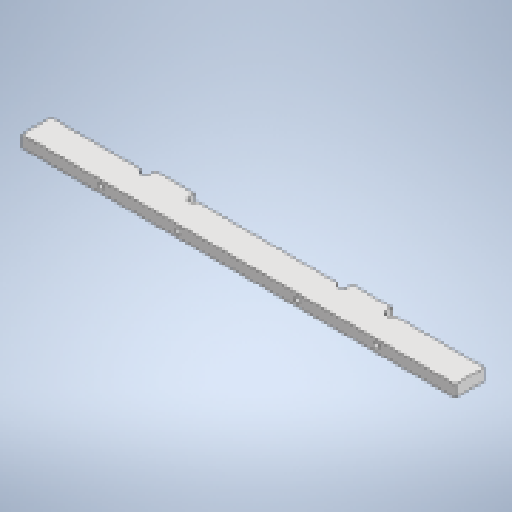
# Autodesk Inventor part: wall
Saved by Autodesk Inventor 2024 (Build 280153000, 153)
## iProperties
Created: 2024-06-06
Part Number: wall
Material: 一般
Document SubType Name: Modeling
Designer: right
Density: 1 g/cm^3
Appearance: 既定
Author: right
Autodesk Inventor part; units mm, degrees
ref_plane "YZ Plane" through (0, 0, 0) normal (1, 0, 0) x (0, 1, 0)
ref_plane "XZ Plane" through (0, 0, 0) normal (0, 1, 0) x (-1, 0, 0)
ref_plane "XY Plane" through (0, 0, 0) normal (0, 0, 1) x (1, 0, 0)
sketch "スケッチ1" plane through (0, 0, 0) normal (0, 0, 1) x (1, 0, 0)
  line L0 (55.5, 22.0883) -> (-55.5, 22.0883)
  line L1 (-55.5, 22.0883) -> (-55.5, 25.0883)
  line L2 (-55.5, 25.0883) -> (55.5, 25.0883)
  line L3 (55.5, 25.0883) -> (55.5, 22.0883)
  line L4 (-22.45, 22.0883) -> (-28.05, 22.0883) projected
  point P0 (0, 0)
  point P1 (-55.5, 26.1052)
  dimension "d0" = 3
  dimension "d1" = 111
  constraints: 8 end point, 2 parallel, 1 horizontal, 1 perpendicular, 1 point on line, 1 vertical alignment, 1 other
  measures "d0" distance of L0.end L1.end
  measures "d1" distance of L1.end L2.end
ref_plane "作業平面1" through (1.2806, -38.0265, 7.5) normal (0, 0, 1) x (0.824865, -0.5653297, 0)
extrude "押し出し1" add sketch "スケッチ1" along normal up to surface (7.5 mm away)
sketch "スケッチ2" plane through (0, 0, 0) normal (0, 0, -1) x (-1, 0, 0)
  line L0 (30.25, 26.1052) -> (30.25, 22.0883) projected
  line L1 (20.25, 22.0883) -> (20.25, 26.1052) projected
  line L2 (-20.25, 26.1052) -> (-20.25, 22.0883) projected
  line L3 (-30.25, 22.0883) -> (-30.25, 26.1052) projected
  line L4 (-55.5, 25.0883) -> (55.5, 25.0883) projected
  line L5 (30.25, 22.0883) -> (20.25, 22.0883)
  line L6 (20.25, 22.0883) -> (20.25, 25.0883)
  line L7 (20.25, 25.0883) -> (30.25, 25.0883)
  line L8 (30.25, 25.0883) -> (30.25, 22.0883)
  line L9 (-20.25, 22.0883) -> (-30.25, 22.0883)
  line L10 (-30.25, 22.0883) -> (-30.25, 25.0883)
  line L11 (-30.25, 25.0883) -> (-20.25, 25.0883)
  line L12 (-20.25, 25.0883) -> (-20.25, 22.0883)
  point P0 (0, 0)
  point P1 (-20.25, 25.0883)
  point P2 (30.25, 25.0883)
  constraints: 16 end point, 4 parallel, 4 point on line, 2 horizontal, 2 perpendicular
ref_plane "作業平面2" through (-55.5, -26.1052, -1.5) normal (0, 0, -1) x (0, 1, 0)
extrude "押し出し2" add sketch "スケッチ2" along normal up to surface (1.5 mm away)
sketch "スケッチ3" plane through (-55.5, 25.0883, 7.5) normal (0, 1, 0) x (1, 0, 0)
  line L0 (85.75, 7.5) -> (111, 7.5) projected
  circle A0 centre (86.85, 7.5) radius 1.1
  line L1 (85.75, 7.5) -> (85.75, 9) projected
  line L2 (75.75, 7.5) -> (35.25, 7.5) projected
  circle A1 centre (74.65, 7.5) radius 1.1
  line L3 (75.75, 7.5) -> (75.75, 9) projected
  line L4 (35.25, 9) -> (35.25, 7.5) projected
  line L5 (25.25, 7.5) -> (25.25, 9) projected
  line L6 (0, 7.5) -> (25.25, 7.5) projected
  circle A2 centre (36.35, 7.5) radius 1.1
  circle A3 centre (24.15, 7.5) radius 1.1
  point P0 (55.5, 7.5)
  dimension "d6" = 2.2
  dimension "d7" = 2.2
  dimension "d8" = 2.2
  dimension "d9" = 2.2
  constraints: 3 horizontal alignment, 3 point on line, 2 vertical, 1 centre point, 1 tangent, 6 other
  measures "d9" diameter of A3
extrude "押し出し3" cut sketch "スケッチ3" against normal through all
sketch "スケッチ4" plane through (0, 0, 0) normal (0, 0, -1) x (-1, 0, 0)
  circle A0 centre (-35.25, 23.5883) radius 1.1 projected
  circle A1 centre (-15.25, 23.5883) radius 1.1 projected
  circle A2 centre (15.25, 23.5883) radius 1.1 projected
  circle A3 centre (35.25, 23.5883) radius 1.1 projected
  point P0 (0, 0)
  constraints: 4 coincident
hole "穴1" at (35.25, 23.5883, 0) at (15.25, 23.5883, 0) at (-15.25, 23.5883, 0) at (-35.25, 23.5883, 0) direction (0, 0, 1) diameter 1.567 end through all thread size "M2x0.4" class "6H" standard "ISO Metric profile"
sketch "スケッチ5" plane through (-55.5, 25.0883, 7.5) normal (0, 1, 0) x (1, 0, 0)
  arc A0 (35.25, 7.5) -> (37.45, 7.5) centre (36.35, 7.5) ccw projected
  line L0 (35.25, 7.5) -> (35.25, 9) projected
  line L1 (35.25, 9) -> (25.25, 9) projected
  line L2 (25.25, 7.5) -> (25.25, 9) projected
  arc A1 (23.05, 7.5) -> (25.25, 7.5) centre (24.15, 7.5) ccw projected
  line L3 (23.05, 7.5) -> (0, 7.5) projected
  line L4 (0, 7.5) -> (0, 0) projected
  line L5 (0, 0) -> (111, 0) projected
  line L6 (111, 7.5) -> (111, 0) projected
  line L7 (111, 7.5) -> (87.95, 7.5) projected
  arc A2 (85.75, 7.5) -> (87.95, 7.5) centre (86.85, 7.5) ccw projected
  line L8 (85.75, 7.5) -> (85.75, 9) projected
  line L9 (85.75, 9) -> (75.75, 9) projected
  line L10 (75.75, 7.5) -> (75.75, 9) projected
  arc A3 (73.55, 7.5) -> (75.75, 7.5) centre (74.65, 7.5) ccw projected
  line L11 (73.55, 7.5) -> (37.45, 7.5) projected
  line L12 (111, 3.75) -> (0, 3.75) construction
  arc A4 (37.45, 0) -> (35.25, 0) centre (36.35, 0) ccw
  line L13 (35.25, 0) -> (35.25, -1.5)
  line L14 (35.25, -1.5) -> (25.25, -1.5)
  line L15 (25.25, 0) -> (25.25, -1.5)
  arc A5 (25.25, 0) -> (23.05, 0) centre (24.15, 0) ccw
  arc A6 (87.95, 0) -> (85.75, 0) centre (86.85, 0) ccw
  line L16 (85.75, 0) -> (85.75, -1.5)
  line L17 (85.75, -1.5) -> (75.75, -1.5)
  line L18 (75.75, 0) -> (75.75, -1.5)
  arc A7 (75.75, 0) -> (73.55, 0) centre (74.65, 0) ccw
  point P0 (55.5, 7.5)
  point P1 (35.25, 0)
  point P2 (23.05, 0)
  point P3 (35.25, 0)
  constraints: 16 symmetric about line, 14 end point, 8 point on circle, 4 centre point, 2 midpoint, 4 other
extrude "押し出し4" add sketch "スケッチ5" against normal up to surface (3 mm away) contours L5 L13 L14 L15 | L16 L17 L18 L5
extrude "押し出し5" cut sketch "スケッチ5" against normal through all contours A5 L5 | A4 L5 | L5 A6 | A7 L5
